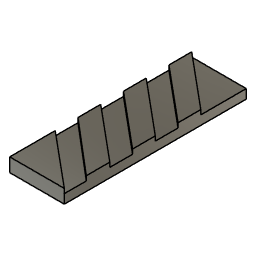
Chaussette (Autodesk Fusion 360 design; units mm, degrees)
Autodesk Fusion 360 part; units mm, degrees
sketch "Sketch1" plane through (0, 0, 0) normal (0, 0, 1) x (1, 0, 0)
  line L0 (0, 0) -> (6, 0)
  line L1 (6, 0) -> (6, 20)
  line L2 (6, 20) -> (0, 20)
  line L3 (0, 20) -> (0, 0)
  dimension "d1" = 6
  dimension "d2" = 20
  constraint horizontal L0
  constraint vertical L1
  constraint horizontal L2
  constraint vertical L3
  constraint coincident L0.start L3.end
  measures "d1" distance of L0.start L0.end
  measures "d2" distance of L0.start L2.end
extrude "Extrude1" add sketch "Sketch1" along normal blind 1 makes body 1
sketch "Sketch2" plane through (0, 0, 1) normal (0, 0, 1) x (-1, 0, 0)
  line L0 (0, -20) -> (0, 0)
  line L1 (0, 0) -> (-6, 0)
  line L2 (-6, 0) -> (-6, -20)
  line L3 (-6, -20) -> (0, -20)
  line L4 (0, -20) -> (-6, -15)
  line L5 (0, -15) -> (-6, -10)
  line L6 (0, -10) -> (-6, -5)
  line L7 (0, -5) -> (-6, 0)
  line L8 (0, -7.5) -> (-6, -2.4178)
  line L9 (0, -12.5) -> (-6, -7.5)
  line L10 (0, -17.5) -> (-6, -12.5)
  constraint coincident L0.start L3.end
  constraint coincident L2 L4.end
  constraint coincident L0 L5.start
  constraint midpoint L2 L5.end
  constraint midpoint L0 L6.start
  constraint coincident L2 L6.end
  constraint parallel L5 L6
  constraint coincident L0 L7.start
  constraint coincident L1.end L2.start
  constraint coincident L0 L8.start
  constraint coincident L2 L8.end
  constraint coincident L0 L9.start
  constraint coincident L2 L9.end
  constraint coincident L2 L10.end
  constraint parallel L5 L10
extrude "Extrude2" add sketch "Sketch2" along normal blind 0.5 contours L0 L2 L4 L10 | L0 L2 L5 L9 | L0 L2 L6 L8 | L0 L1 L7 bodies 1
copy_body "Body->Comp1" bodies 1 removing the originals makes body 2 in component "Component"
component "Component" placed x (1, 0, 0) y (0, 1, 0) z (0, 0, 1) at (0, 0, 0)
